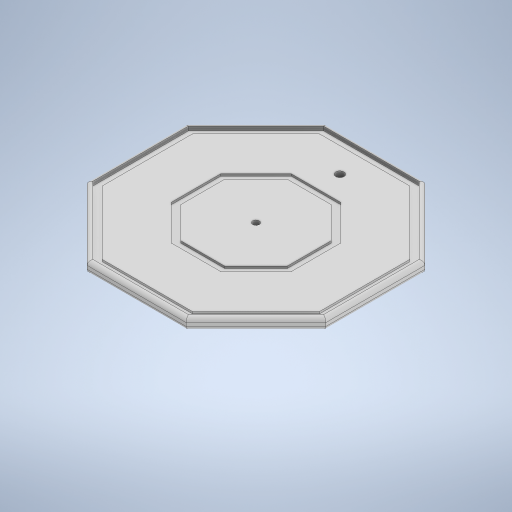
# Autodesk Inventor part: OV-PAM_top_2
Saved by Autodesk Inventor 2024 (Build 280153000, 153)
## iProperties
Created: 2023-06-16
Part Number: OV-PAM_top_2
Material: 일반
Document SubType Name: Modeling
Designer: jsw
Density: 1 g/cm^3
Appearance: 기본값
Author: jsw
Autodesk Inventor part; units mm, degrees
ref_plane "YZ Plane" through (0, 0, 0) normal (1, 0, 0) x (0, 1, 0)
ref_plane "XZ Plane" through (0, 0, 0) normal (0, 1, 0) x (-1, 0, 0)
ref_plane "XY Plane" through (0, 0, 0) normal (0, 0, 1) x (1, 0, 0)
sketch "스케치3" plane through (0, 0, 0) normal (0, 1, 0) x (-1, 0, 0)
  line L0 (35.5919, -14.7426) -> (14.7426, -35.5919)
  line L1 (14.7426, -35.5919) -> (-14.7426, -35.5919)
  line L2 (-14.7426, -35.5919) -> (-35.5919, -14.7426)
  line L3 (-35.5919, -14.7426) -> (-35.5919, 14.7426)
  line L4 (-35.5919, 14.7426) -> (-14.7426, 35.5919)
  line L5 (-14.7426, 35.5919) -> (14.7426, 35.5919)
  line L6 (14.7426, 35.5919) -> (35.5919, 14.7426)
  line L7 (35.5919, 14.7426) -> (35.5919, -14.7426)
  line L8 (32.5919, -13.5) -> (13.5, -32.5919)
  line L9 (13.5, -32.5919) -> (-13.5, -32.5919)
  line L10 (-13.5, -32.5919) -> (-32.5919, -13.5)
  line L11 (-32.5919, -13.5) -> (-32.5919, 13.5)
  line L12 (-32.5919, 13.5) -> (-13.5, 32.5919)
  line L13 (-13.5, 32.5919) -> (13.5, 32.5919)
  line L14 (13.5, 32.5919) -> (32.5919, 13.5)
  line L15 (32.5919, 13.5) -> (32.5919, -13.5)
  point P0 (0, 0)
  point P1 (0, 0)
  point P2 (0, 0)
  point P3 (0, 0)
  dimension "d43" = 27
  dimension "d44" = 3
  constraints: 32 end point, 3 coincident, 2 horizontal, 34 other
  measures "d43" distance of L8.end L9.end
  measures "d44" distance between parallel lines of L7 L15
extrude "돌출2" add sketch "스케치3" along normal blind 3.4 contours L0 L1 L2 L3 L4 L5 L6 L7 | L8 L9 L10 L11 L12 L13 L14 L15
sketch "스케치4" plane through (0, 3.4, 0) normal (0, 1, 0) x (1, 0, 0)
  line L0 (13.5, -32.5919) -> (-13.5, -32.5919)
  line L1 (-13.5, -32.5919) -> (-32.5919, -13.5)
  line L2 (-32.5919, -13.5) -> (-32.5919, 13.5)
  line L3 (-32.5919, 13.5) -> (-13.5, 32.5919)
  line L4 (-13.5, 32.5919) -> (13.5, 32.5919)
  line L5 (13.5, 32.5919) -> (32.5919, 13.5)
  line L6 (32.5919, 13.5) -> (32.5919, -13.5)
  line L7 (32.5919, -13.5) -> (13.5, -32.5919)
  line L8 (-14.2456, 34.3919) -> (14.2456, 34.3919)
  line L9 (14.2456, 34.3919) -> (34.3919, 14.2456)
  line L10 (34.3919, 14.2456) -> (34.3919, -14.2456)
  line L11 (34.3919, -14.2456) -> (14.2456, -34.3919)
  line L12 (14.2456, -34.3919) -> (-14.2456, -34.3919)
  line L13 (-14.2456, -34.3919) -> (-34.3919, -14.2456)
  line L14 (-34.3919, -14.2456) -> (-34.3919, 14.2456)
  line L15 (-34.3919, 14.2456) -> (-14.2456, 34.3919)
  line L16 (-13.4172, 32.3919) -> (13.4172, 32.3919)
  line L17 (13.4172, 32.3919) -> (32.3919, 13.4172)
  line L18 (32.3919, 13.4172) -> (32.3919, -13.4172)
  line L19 (32.3919, -13.4172) -> (13.4172, -32.3919)
  line L20 (13.4172, -32.3919) -> (-13.4172, -32.3919)
  line L21 (-13.4172, -32.3919) -> (-32.3919, -13.4172)
  line L22 (-32.3919, -13.4172) -> (-32.3919, 13.4172)
  line L23 (-32.3919, 13.4172) -> (-13.4172, 32.3919)
  point P0 (0, 0)
  point P1 (0, 0)
  point P2 (0, 0)
  point P3 (0, 0)
  dimension "d7" = 27
  dimension "d42" = 1.8
  dimension "d45" = 0.2
  constraints: 48 end point, 3 coincident, 3 horizontal, 51 other
  measures "d7" distance of L1.end L2.end
  measures "d42" distance between parallel lines of L14 L2
  measures "d45" distance between parallel lines of L22 L2
extrude "돌출3" cut sketch "스케치4" against normal blind 1.2 contours L0 L1 L2 L3 L4 L5 L6 L7 | L8 L9 L10 L11 L12 L13 L14 L15 | L16 L17 L18 L19 L20 L21 L22 L23
sketch "스케치5" plane through (0, 0, 0) normal (0, -1, 0) x (1, 0, 0)
  line L0 (10, 2.5) -> (20, 2.5)
  line L1 (20, 2.5) -> (20, -2.5)
  line L2 (20, -2.5) -> (10, -2.5)
  line L3 (10, -2.5) -> (10, 2.5)
  line L4 (10, 2.5) -> (20, -2.5) construction
  line L5 (20, 2.5) -> (10, -2.5) construction
  line L6 (-20, 2.5) -> (-10, 2.5)
  line L7 (-10, 2.5) -> (-10, -2.5)
  line L8 (-10, -2.5) -> (-20, -2.5)
  line L9 (-20, -2.5) -> (-20, 2.5)
  line L10 (-20, 2.5) -> (-10, -2.5) construction
  line L11 (-10, 2.5) -> (-20, -2.5) construction
  point P0 (0, 0)
  point P1 (15, 0)
  point P2 (-15, 0)
  dimension "d11" = 10
  dimension "d12" = 5
  dimension "d13" = 10
  dimension "d16" = 30
  constraints: 24 end point, 2 horizontal, 2 midpoint, 2 parallel, 1 collinear, 1 horizontal alignment, 1 perpendicular, 10 other
  measures "d11" distance of L1.end L2.end
  measures "d12" distance of L0.end L1.end
  measures "d13" distance from line of L3 point (0, 0)
  measures "d16" distance of L0.start L6.start
extrude "돌출4" add sketch "스케치5" along normal blind 10
sketch "스케치6" plane through (-10, 0, -2.5) normal (0, 0, -1) x (-1, 0, 0)
  circle A0 centre (5, -10) radius 5
  circle A1 centre (-25, -10) radius 5
  line L0 (-20, -10) -> (-30, -10) projected
  line L1 (10, -10) -> (0, -10) projected
  point P0 (-10, 0)
  dimension "d23" = 10
  dimension "d24" = 10
  constraints: 2 centre point, 2 coincident, 2 midpoint
  measures "d23" diameter of A0
  measures "d24" diameter of A1
extrude "돌출5" add sketch "스케치6" against normal blind 5
sketch "스케치7" plane through (-10, 0, -2.5) normal (0, 0, -1) x (-1, 0, 0)
  circle A0 centre (5, -10) radius 1.25
  line L0 (10, 0) -> (10, -10) projected
  line L1 (0, 0) -> (10, 0) projected
  line L2 (4.7788, 0) -> (0, 0)
  circle A1 centre (-25, -10) radius 1.25
  point P0 (-10, 0)
  dimension "d27" = 2.5
  dimension "d28" = 5
  dimension "d31" = 30
  constraints: 2 centre point, 2 end point, 1 horizontal, 1 horizontal alignment, 1 point on line, 2 other
  measures "d27" diameter of A0
  measures "d28" distance from line of L0 A0.centre
  measures "d31" distance of A0.centre A1.centre
extrude "돌출6" cut sketch "스케치7" against normal blind 5
sketch "스케치8" plane through (0, 0, 0) normal (0, -1, 0) x (1, 0, 0)
  circle A0 centre (0, -25) radius 1.25
  line L0 (-10, 2.5) -> (-10, -2.5) projected
  point P0 (0, 0)
  point P1 (-10, 0)
  dimension "d38" = 2.5
  dimension "d39" = 25
  constraints: 1 centre point, 1 midpoint, 1 vertical alignment
  measures "d38" diameter of A0
  measures "d39" vertical distance of A0.centre point (-10, 0)
sketch "스케치9" plane through (0, 2.2, 0) normal (0, 1, 0) x (1, 0, 0)
  line L0 (-13.4172, 32.3919) -> (13.4172, 32.3919)
  line L1 (13.4172, 32.3919) -> (32.3919, 13.4172)
  line L2 (32.3919, 13.4172) -> (32.3919, -13.4172)
  line L3 (32.3919, -13.4172) -> (13.4172, -32.3919)
  line L4 (13.4172, -32.3919) -> (-13.4172, -32.3919)
  line L5 (-13.4172, -32.3919) -> (-32.3919, -13.4172)
  line L6 (-32.3919, -13.4172) -> (-32.3919, 13.4172)
  line L7 (-32.3919, 13.4172) -> (-13.4172, 32.3919)
  line L8 (-14.2456, 34.3919) -> (14.2456, 34.3919) projected
  line L9 (-12.1745, 29.3919) -> (12.1745, 29.3919)
  line L10 (12.1745, 29.3919) -> (29.3919, 12.1745)
  line L11 (29.3919, 12.1745) -> (29.3919, -12.1745)
  line L12 (29.3919, -12.1745) -> (12.1745, -29.3919)
  line L13 (12.1745, -29.3919) -> (-12.1745, -29.3919)
  line L14 (-12.1745, -29.3919) -> (-29.3919, -12.1745)
  line L15 (-29.3919, -12.1745) -> (-29.3919, 12.1745)
  line L16 (-29.3919, 12.1745) -> (-12.1745, 29.3919)
  point P0 (0, 0)
  point P1 (0, 0)
  point P2 (0, 0)
  dimension "d46" = 2
  dimension "d47" = 3
  constraints: 32 end point, 2 coincident, 2 horizontal, 34 other
  measures "d46" distance between parallel lines of L0 L8
  measures "d47" distance between parallel lines of L0 L9
extrude "돌출8" add sketch "스케치9" along normal blind 0.6 contours L0 L1 L2 L3 L4 L5 L6 L7 | L9 L10 L11 L12 L13 L14 L15 L16
fillet "모깎기1" radius 1.2 16 edges at (-35.5919, 3.4, 0) (-25.1673, 3.4, 25.1673) (0, 3.4, 35.5919) (25.1673, 3.4, 25.1673) (35.5919, 3.4, 0) (25.1673, 3.4, -25.1673) (0, 3.4, -35.5919) (-25.1673, 3.4, -25.1673) (25.1673, 0, 25.1673) (0, 0, 35.5919) (-25.1673, 0, 25.1673) (-35.5919, 0, 0) (-25.1673, 0, -25.1673) (0, 0, -35.5919) (25.1673, 0, -25.1673) (35.5919, 0, 0)
sketch "스케치10" plane through (0, 0, 0) normal (0, -1, 0) x (1, 0, 0)
  line L0 (-20, 2.5) -> (-10, 2.5) projected
  line L1 (-10, -2.5) -> (-20, -2.5) projected
  line L2 (-20, 2.5) -> (-19, 2.5)
  line L3 (-19, 2.5) -> (-19, -2.5)
  line L4 (-19, -2.5) -> (-20, -2.5)
  line L5 (-20, -2.5) -> (-20, 2.5)
  line L6 (20, -2.5) -> (10, -2.5) projected
  line L7 (10, 2.5) -> (20, 2.5) projected
  line L8 (20, -2.5) -> (19, -2.5)
  line L9 (19, -2.5) -> (19, 2.5)
  line L10 (19, 2.5) -> (20, 2.5)
  line L11 (20, 2.5) -> (20, -2.5)
  point P0 (0, 0)
  dimension "d54" = 1
  dimension "d55" = 1
  constraints: 16 end point, 4 parallel, 2 horizontal, 2 perpendicular, 2 point on line
  measures "d54" distance of L1.end L3.end
  measures "d55" distance of L9.end L10.end
extrude "돌출9" cut sketch "스케치10" along normal blind 15
extrude "돌출10" cut sketch "스케치8" against normal blind 5
sketch "스케치11" plane through (0, 2.8, 0) normal (0, 1, 0) x (1, 0, 0)
  line L0 (-6.575, 15.8735) -> (6.575, 15.8735)
  line L1 (6.575, 15.8735) -> (15.8735, 6.575)
  line L2 (15.8735, 6.575) -> (15.8735, -6.575)
  line L3 (15.8735, -6.575) -> (6.575, -15.8735)
  line L4 (6.575, -15.8735) -> (-6.575, -15.8735)
  line L5 (-6.575, -15.8735) -> (-15.8735, -6.575)
  line L6 (-15.8735, -6.575) -> (-15.8735, 6.575)
  line L7 (-15.8735, 6.575) -> (-6.575, 15.8735)
  line L8 (-7.4034, 17.8735) -> (7.4034, 17.8735)
  line L9 (7.4034, 17.8735) -> (17.8735, 7.4034)
  line L10 (17.8735, 7.4034) -> (17.8735, -7.4034)
  line L11 (17.8735, -7.4034) -> (7.4034, -17.8735)
  line L12 (7.4034, -17.8735) -> (-7.4034, -17.8735)
  line L13 (-7.4034, -17.8735) -> (-17.8735, -7.4034)
  line L14 (-17.8735, -7.4034) -> (-17.8735, 7.4034)
  line L15 (-17.8735, 7.4034) -> (-7.4034, 17.8735)
  point P0 (0, 0)
  point P1 (0, 0)
  point P2 (0, 0)
  point P3 (0, 17.8735)
  dimension "d60" = 13.15
  dimension "d61" = 2
  constraints: 32 end point, 2 coincident, 2 horizontal, 1 midpoint, 34 other
  measures "d60" distance of L5.end L6.end
  measures "d61" distance between parallel lines of L6 L14
extrude "돌출11" cut sketch "스케치11" against normal blind 0.6
sketch "스케치12" plane through (0, 2.8, 0) normal (0, 1, 0) x (1, 0, 0)
  circle A0 centre (0, 0) radius 1
  dimension "d64" = 2
  constraints: 1 centre point, 1 coincident
  measures "d64" diameter of A0
extrude "돌출12" cut sketch "스케치12" against normal up to surface (2.8 mm away)
equation "\"d55\" = d54"
